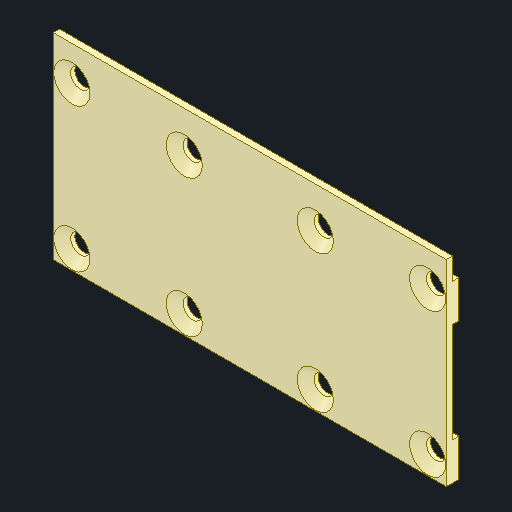
# Autodesk Inventor part: back
Saved by Autodesk Inventor 2023 (Build 270158000, 158)
## iProperties
Created: 2024-05-19
Part Number: back
Material: Nylon 6/6
Document SubType Name: Modeling
Designer: szymo
Density: 1.13 g/cm^3
Appearance: Nylon 6
Mass: 3.25364 g
Surface Area: 45.9491 cm^2
Volume: 2.87933 cm^3
Author: szymo
Autodesk Inventor part; units mm, degrees
ref_plane "YZ Plane" through (0, 0, 0) normal (1, 0, 0) x (0, 1, 0)
ref_plane "XZ Plane" through (0, 0, 0) normal (0, 1, 0) x (-1, 0, 0)
ref_plane "XY Plane" through (0, 0, 0) normal (0, 0, 1) x (1, 0, 0)
ref_plane "Work Plane1" through (22, 31.5, 0) normal (0, 0, 1) x (0, 1, 0)
sketch "Sketch1" plane through (22, 31.5, 0) normal (0, 0, 1) x (0, 1, 0)
  line L0 (0, 0) -> (0, 61) projected
  line L1 (0, 61) -> (-3.5, 61) projected
  line L2 (-3.5, 0) -> (-3.5, 61) projected
  circle A0 centre (-5.5, 2) radius 1.75 projected
  circle A1 centre (-28.5, 2) radius 1.75 projected
  line L3 (-3.5, 4) -> (-7.5, 4) projected
  arc A2 (-8.5, 3) -> (-7.5, 4) centre (-8.5, 4) ccw projected
  line L4 (-8.5, 3) -> (-21.7679, 3) projected
  arc A3 (-23.5, 4) -> (-21.7679, 3) centre (-21.7679, 5) ccw projected
  line L5 (-23.5, 4) -> (-31.5, 4) projected
  line L6 (-31.5, 0) -> (-31.5, 4) projected
  line L7 (-3.5, 0) -> (-3.5, 4) projected
  line L8 (-31.5, 22) -> (-3.5, 22) projected
  line L9 (-31.5, 22) -> (-31.5, 18) projected
  line L10 (-3.5, 22) -> (-3.5, 18) projected
  line L11 (-31.5, 39) -> (-3.5, 39) projected
  line L12 (-3.5, 39) -> (-3.5, 43) projected
  line L13 (-31.5, 39) -> (-31.5, 43) projected
  line L14 (-3.5, 57) -> (-6.7679, 57) projected
  line L15 (-3.5, 61) -> (-3.5, 57) projected
  line L16 (-3.5, 61) -> (-31.5, 61) projected
  line L17 (-31.5, 61) -> (-31.5, 57) projected
  line L18 (-24.004, 57) -> (-31.5, 57) projected
  line L19 (0, -1) -> (-31.5, -1)
  line L20 (-31.5, -1) -> (-31.5, 62)
  line L21 (-31.5, 62) -> (0, 62)
  line L22 (0, 62) -> (0, -1)
  line L23 (-3.5, 0) -> (-31.5, 0)
  circle A4 centre (-28.5, 20) radius 1.75 projected
  circle A5 centre (-28.5, 41) radius 1.75 projected
  circle A6 centre (-6.5, 41) radius 1.75 projected
  line L24 (-31.5, 43) -> (-3.5, 43) projected
  line L25 (-8.5, 58) -> (-21.7679, 58) projected
  arc A7 (-7.634, 57.5) -> (-6.7679, 57) centre (-6.7679, 58) ccw projected
  arc A8 (-24.004, 57) -> (-23.2587, 57.3333) centre (-24.004, 58) ccw projected
  arc A9 (-21.7679, 58) -> (-23.2587, 57.3333) centre (-21.7679, 56) ccw projected
  arc A10 (-7.634, 57.5) -> (-8.5, 58) centre (-8.5, 57) ccw projected
  circle A11 centre (-6.5, 20) radius 1.75 projected
  line L26 (-31.5, 18) -> (-3.5, 18) projected
  circle A12 centre (-5.5, 59) radius 1.75 projected
  circle A13 centre (-28.5, 59) radius 1.75 projected
  point P0 (-3.5, 28.5)
  point P1 (-3.5, 32.5)
  point P2 (-3.5, 61)
  point P3 (-13.5, 58)
  point P4 (-27.0639, 40)
  point P5 (-29.9361, 40)
  point P6 (-27.0639, 21)
  point P7 (-29.9361, 21)
  dimension "d25" = 1
  dimension "d26" = 1
  constraints: 10 end point, 1 collinear, 1 horizontal, 1 parallel, 1 perpendicular, 1 vertical, 1 other
  measures "d25" distance between parallel lines of L21 L1
  measures "d26" distance from line of point (-3.5, 0) L19
extrude "Extrusion1" add sketch "Sketch1" along normal blind 2 contours L22 L19 L20 L23 L2 L1 L0 | L1 L16 L20 L21 L22 | L2 L14 A7 A10 L25 A9 A8 L18 L17 L16 | L2 L24 L20 L18 A8 A9 L25 A10 A7 L14 | L6 L5 A3 L4 A2 L3 L2 L23 | L2 L11 L13 L24 | L20 L26 L2 L3 A2 L4 A3 L5 | L2 L8 L20 L11 | L9 L8 L2 L26 | A0 | A1 | A4 | A5 | A6 | A11 | A12 | A13
sketch "Sketch2" plane through (22, 31.5, 2) normal (0, 0, 1) x (1, 0, 0)
  circle A0 centre (-2, -5.5) radius 1.75 projected
  circle A1 centre (-2, -28.5) radius 1.75 projected
  circle A2 centre (-20, -6.5) radius 1.75 projected
  circle A3 centre (-59, -28.5) radius 1.75 projected
  circle A4 centre (-59, -5.5) radius 1.75 projected
  circle A5 centre (-41, -28.5) radius 1.75 projected
  circle A6 centre (-20, -28.5) radius 1.75 projected
  circle A7 centre (-41, -6.5) radius 1.75 projected
  point P0 (-22, -31.5)
  point P1 (-40, -5.0639)
  point P2 (-40, -7.9361)
  point P3 (-40, -27.0639)
  point P4 (-40, -29.9361)
  point P5 (-21, -27.0639)
  point P6 (-21, -29.9361)
  constraints: 5 coincident
hole "Hole1" at (20, 3, 2) at (20, 26, 2) at (2, 25, 2) at (2, 3, 2) at (-19, 3, 2) at (-19, 25, 2) at (-37, 26, 2) at (-37, 3, 2) direction (0, 0, -1) diameter 3.1 end through all countersink diameter 5.8 countersink angle 90 clearance for "Countersunk Flat Head Screw ISO 2009/7046" size "M2.5" standard "ISO"
sketch "Sketch3" plane through (22, 31.5, 0) normal (0, 0, -1) x (-1, 0, 0)
  line L0 (4, -3.5) -> (4, -6.7679) projected
  arc A0 (3, -21.7679) -> (3.6667, -23.2587) centre (5, -21.7679) ccw projected
  line L1 (4, -24.004) -> (4, -31.5) projected
  line L2 (0, -31.5) -> (4, -31.5) projected
  line L3 (0, -3.5) -> (0, -31.5) projected
  line L4 (0, -3.5) -> (4, -3.5) projected
  line L5 (22, -31.5) -> (22, -3.5) projected
  line L6 (22, -31.5) -> (18, -31.5) projected
  line L7 (22, -3.5) -> (18, -3.5) projected
  line L8 (39, -31.5) -> (39, -3.5) projected
  line L9 (39, -3.5) -> (43, -3.5) projected
  line L10 (39, -31.5) -> (43, -31.5) projected
  line L11 (57, -3.5) -> (57, -6.7679) projected
  line L12 (61, -3.5) -> (57, -3.5) projected
  line L13 (61, -3.5) -> (61, -31.5) projected
  line L14 (61, -31.5) -> (57, -31.5) projected
  line L15 (57, -24.004) -> (57, -31.5) projected
  line L16 (62, -31.5) -> (-1, -31.5)
  line L17 (-1, -31.5) -> (-1, -25.5)
  line L18 (-1, -25.5) -> (62, -25.5)
  line L19 (62, -25.5) -> (62, -31.5)
  circle A1 centre (59, -5.5) radius 1.55 projected
  circle A2 centre (41, -28.5) radius 1.55 projected
  circle A3 centre (20, -6.5) radius 1.55 projected
  circle A4 centre (2, -28.5) radius 1.55 projected
  circle A5 centre (2, -5.5) radius 1.55 projected
  circle A6 centre (20, -28.5) radius 1.55 projected
  circle A7 centre (41, -6.5) radius 1.55 projected
  circle A8 centre (59, -28.5) radius 1.55 projected
  line L20 (-1, 0) -> (62, 0) projected
  line L21 (62, -9.5) -> (-1, -9.5)
  line L22 (-1, -9.5) -> (-1, -3.5)
  line L23 (-1, -3.5) -> (62, -3.5)
  line L24 (62, -3.5) -> (62, -9.5)
  circle A9 centre (59, -28.5) radius 1.55 projected
  circle A10 centre (41, -6.5) radius 1.55 projected
  line L25 (59, -28.5) -> (41, -6.5) construction
  circle A11 centre (41, -28.5) radius 1.55 projected
  line L26 (59, -5.5) -> (41, -28.5) construction
  line L27 (41, -28.5) -> (20, -6.5) construction
  circle A12 centre (2, -28.5) radius 1.55 projected
  line L28 (20, -6.5) -> (2, -28.5) construction
  circle A13 centre (2, -5.5) radius 1.55 projected
  line L29 (2, -5.5) -> (20, -28.5) construction
  line L30 (20, -28.5) -> (41, -6.5) construction
  line L31 (54.6074, -25.5) -> (41.5165, -9.5)
  line L32 (45.3926, -9.5) -> (58.4835, -25.5)
  line L33 (57.7743, -9.5) -> (45.2526, -25.5)
  line L34 (41.4431, -25.5) -> (53.9648, -9.5)
  line L35 (40.21, -9.5) -> (24.9373, -25.5)
  line L36 (20.79, -25.5) -> (36.0627, -9.5)
  line L37 (19.4835, -9.5) -> (6.3926, -25.5)
  line L38 (2.5165, -25.5) -> (15.6074, -9.5)
  line L39 (40.21, -25.5) -> (24.9373, -9.5)
  line L40 (20.79, -9.5) -> (36.0627, -25.5)
  line L41 (19.5569, -25.5) -> (7.0352, -9.5)
  line L42 (3.2257, -9.5) -> (15.7474, -25.5)
  line L43 (62, -25.5) -> (57.7743, -25.5)
  line L44 (57.7743, -25.5) -> (57.7743, -9.5)
  line L45 (57.7743, -9.5) -> (62, -9.5)
  line L46 (62, -9.5) -> (62, -25.5)
  line L47 (-1, -25.5) -> (3.2257, -25.5)
  line L48 (3.2257, -25.5) -> (3.2257, -9.5)
  line L49 (3.2257, -9.5) -> (-1, -9.5)
  line L50 (-1, -9.5) -> (-1, -25.5)
  line L51 (62, 0) -> (62, -31.5) projected
  line L52 (-1, -31.5) -> (-1, 0) projected
  line L53 (62, -31.5) -> (-1, -31.5) projected
  line L54 (3, -8.5) -> (3, -21.7679) projected
  arc A14 (3.5, -7.634) -> (4, -6.7679) centre (3, -6.7679) ccw projected
  arc A15 (3.5, -7.634) -> (3, -8.5) centre (4, -8.5) ccw projected
  arc A16 (4, -24.004) -> (3.6667, -23.2587) centre (3, -24.004) ccw projected
  circle A17 centre (20, -28.5) radius 1.75 projected
  circle A18 centre (41, -28.5) radius 1.75 projected
  circle A19 centre (41, -6.5) radius 1.75 projected
  line L55 (43, -31.5) -> (43, -3.5) projected
  line L56 (58, -8.5) -> (58, -21.7679) projected
  arc A20 (57, -6.7679) -> (57.5, -7.634) centre (58, -6.7679) ccw projected
  arc A21 (57.3333, -23.2587) -> (57, -24.004) centre (58, -24.004) ccw projected
  arc A22 (57.3333, -23.2587) -> (58, -21.7679) centre (56, -21.7679) ccw projected
  arc A23 (58, -8.5) -> (57.5, -7.634) centre (57, -8.5) ccw projected
  circle A24 centre (20, -6.5) radius 1.75 projected
  line L57 (18, -31.5) -> (18, -3.5) projected
  circle A25 centre (2, -5.5) radius 1.75 projected
  circle A26 centre (2, -28.5) radius 1.75 projected
  circle A27 centre (59, -5.5) radius 1.75 projected
  circle A28 centre (59, -28.5) radius 1.75 projected
  point P0 (3.2257, -22.6909)
  point P1 (4, -25.5)
  point P2 (4.978, -23.4871)
  point P3 (9.2789, -17.2347)
  point P4 (11.226, -14.855)
  point P5 (11.174, -19.6561)
  point P6 (28.4263, -17.5)
  point P7 (13.1211, -17.2764)
  point P8 (30.5, -19.6724)
  point P9 (30.5, -15.3276)
  point P10 (49.826, -19.6561)
  point P11 (47.8789, -17.2764)
  point P12 (32.5737, -17.5)
  point P13 (49.774, -14.855)
  point P14 (51.7211, -17.2347)
  point P15 (0, -9.5)
  point P16 (0, -25.5)
  point P17 (4, -25.5)
  point P18 (0, -25.5)
  point P19 (4, -23.6868)
  point P20 (3.2257, -24.6332)
  point P21 (3.2257, -25.5)
  point P22 (61, -9.5)
  point P23 (22, -24.2323)
  point P24 (57, -23.6868)
  point P25 (-1, -3.5)
  point P26 (62, -3.5)
  point P27 (-1, -9.5)
  point P28 (58, -13.5)
  point P29 (40, -27.0639)
  point P30 (40, -29.9361)
  point P31 (21, -27.0639)
  point P32 (21, -29.9361)
  dimension "d9" = 6
  dimension "d10" = 6
  dimension "d11" = 1.5
  dimension "d12" = 1.5
  dimension "d13" = 1.5
  dimension "d14" = 1.5
  dimension "d15" = 1.5
  dimension "d16" = 1.5
  dimension "d17" = 1.5
  dimension "d18" = 1.5
  dimension "d19" = 1.5
  dimension "d20" = 1.5
  dimension "d21" = 1.5
  dimension "d22" = 1.5
  constraints: 64 end point, 18 parallel, 5 horizontal, 3 perpendicular, 2 collinear, 1 point on line, 1 vertical, 30 other
  measures "d9" distance of L16.end L17.end
  measures "d10" distance of L22.start L22.end
  measures "d11" distance between parallel lines of L25 L31
  measures "d12" distance between parallel lines of L32 L25
  measures "d13" distance between parallel lines of L26 L34
  measures "d14" distance between parallel lines of L26 L33
  measures "d15" distance between parallel lines of L30 L35
  measures "d16" distance between parallel lines of L30 L36
  measures "d17" distance between parallel lines of L37 L28
  measures "d18" distance between parallel lines of L28 L38
  measures "d19" distance between parallel lines of L27 L40
  measures "d20" distance between parallel lines of L27 L39
  measures "d21" distance between parallel lines of L29 L41
  measures "d22" distance between parallel lines of L42 L29
extrude "zeberka" cut sketch "Sketch3" against normal blind 1 contours L4 L23 L52 L20 L51 L12 L9 L7 | L21 L54 A0 L48 L38 L18 L3 | L3 L18 L50 L21 | L21 L48 A0 L54 | L21 L40 L5 L36 L18 L41 L57 L37 | L38 L41 L21 | L57 L41 L37 | L42 L38 A16 A0 L48 | L40 L36 L5 | L21 L36 L39 | L48 A0 A16 L38 | L35 L21 L31 L55 L34 L18 L39 L8 | L8 L39 L35 | L42 L18 L37 | L46 L18 L13 L21 | L40 L18 L35 | L21 L34 L32 | L31 L34 L55 | L13 L18 L32 L44 A22 L56 L21 | L56 A22 L44 L21 | L44 A22 A21 L32 L33 | L31 L18 L33 | L44 L32 A21 A22
equation "\"d10\" = d9"
equation "\"d12\" = d11"
equation "\"d13\" = d11"
equation "\"d14\" = d11"
equation "\"d15\" = d11"
equation "\"d16\" = d11"
equation "\"d17\" = d11"
equation "\"d18\" = d11"
equation "\"d19\" = d11"
equation "\"d20\" = d11"
equation "\"d21\" = d11"
equation "\"d22\" = d11"
body "Solid1"
